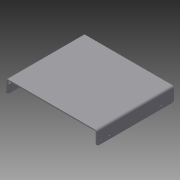
# Autodesk Inventor part: Bed
Saved by Autodesk Inventor 2015 (Build 190159000, 159)
## iProperties
Created: 2015-12-09
Part Number: Bed
Material: Generic
Document SubType Name: Sheet Metal
Designer: Nick
Density: 1 g/cm^3
Flat Pattern Width: 21.3893 cm
Flat Pattern Length: 31.6732 cm
Flat Pattern Area: 677.468 cm^2
Sheet Metal Rule: Default
Sheet Metal Width: 8.421 in
Sheet Metal Length: 12.470 in
Sheet Metal Area: 105.008 in^2
Appearance: Default
Author: Nick
Autodesk Inventor part; units mm, degrees
ref_plane "YZ Plane" through (0, 0, 0) normal (1, 0, 0) x (0, 1, 0)
ref_plane "XZ Plane" through (0, 0, 0) normal (0, 1, 0) x (-1, 0, 0)
ref_plane "XY Plane" through (0, 0, 0) normal (0, 0, 1) x (1, 0, 0)
sketch "Sketch1" plane through (0, 0, 0) normal (0, 1, 0) x (-1, 0, 0)
  line L0 (0, 0) -> (0, -213.8934)
  line L1 (0, -213.8934) -> (236.982, -213.8934)
  line L2 (236.982, -213.8934) -> (236.982, 0)
  line L3 (236.982, 0) -> (0, 0)
  line L4 (246.3292, 0) -> (270.5069, 0)
  line L5 (246.3292, -213.8934) -> (246.3292, 0)
  line L6 (270.5069, 0) -> (270.5069, 0)
  line L7 (276.8569, -6.35) -> (276.8569, -207.5434)
  arc A0 (276.8569, -6.35) -> (270.5069, 0) centre (270.5069, -6.35) ccw
  arc A1 (270.5068, -213.8934) -> (276.8569, -207.5434) centre (270.5069, -207.5434) ccw
  line L8 (236.982, 0) -> (246.3292, 0)
  line L9 (236.982, -213.8934) -> (246.3292, -213.8934)
  line L10 (241.6556, 0) -> (241.6556, -213.8934)
  line L11 (246.3292, -213.8934) -> (270.5068, -213.8934)
  line L12 (118.491, 0) -> (118.491, -213.8934)
  line L13 (0, -213.8934) -> (0, 0)
  line L14 (-9.3472, 0) -> (-33.5249, 0)
  line L15 (-9.3472, -213.8934) -> (-9.3472, 0)
  line L16 (-33.5249, 0) -> (-33.5249, 0)
  line L17 (-39.8749, -6.35) -> (-39.8749, -207.5434)
  arc A2 (-33.5249, 0) -> (-39.8749, -6.35) centre (-33.5249, -6.35) ccw
  arc A3 (-39.8749, -207.5434) -> (-33.5248, -213.8934) centre (-33.5249, -207.5434) ccw
  line L18 (0, 0) -> (-9.3472, 0)
  line L19 (0, -213.8934) -> (-9.3472, -213.8934)
  line L20 (-4.6736, 0) -> (-4.6736, -213.8934)
  line L21 (-9.3472, -213.8934) -> (-33.5248, -213.8934)
  circle A4 centre (267.6621, -35.1028) radius 1.4986
  line L22 (276.8569, -106.9467) -> (236.982, -106.9467)
  circle A5 centre (267.6621, -178.7906) radius 1.4986
  circle A6 centre (-30.6801, -35.1028) radius 1.4986
  circle A7 centre (-30.6801, -178.7906) radius 1.4986
  line L23 (246.9642, -4.4704) -> (249.3518, -4.4704)
  line L24 (249.3518, -4.4704) -> (249.3518, -10.6934)
  line L25 (249.3518, -10.6934) -> (246.9642, -10.6934)
  line L26 (246.9642, -10.6934) -> (246.9642, -4.4704)
  line L27 (249.3518, -4.4704) -> (251.5616, -4.4704)
  line L28 (251.5616, -4.4704) -> (251.5616, -10.6934)
  line L29 (251.5616, -10.6934) -> (253.9492, -10.6934)
  line L30 (253.9492, -10.6934) -> (253.9492, -4.4704)
  line L31 (253.9492, -4.4704) -> (251.5616, -4.4704)
  line L32 (-26.0096, -2.9972) -> (-34.4424, -2.9972)
  line L33 (-34.4424, -2.9972) -> (-34.4424, -4.9276)
  line L34 (-34.4424, -4.9276) -> (-26.0096, -4.9276)
  line L35 (-26.0096, -4.9276) -> (-26.0096, -2.9972)
  line L36 (-34.4424, -10.287) -> (-26.0096, -10.287)
  line L37 (-34.4424, -10.287) -> (-34.4424, -12.2174)
  line L38 (-34.4424, -12.2174) -> (-26.0096, -12.2174)
  line L39 (-26.0096, -12.2174) -> (-26.0096, -10.287)
  point P0 (276.8569, 0)
  point P1 (-39.8749, 0)
  dimension "d1" = 213.8934
  dimension "d2" = 236.982
  dimension "d3" = 24.1776
  dimension "d4" = 6.35
  dimension "d5" = 6.35
  dimension "d6" = 9.3472
  dimension "d7" = 213.8934
  dimension "d8" = 24.1776
  dimension "d11" = 2.9972
  dimension "d12" = 9.1948
  dimension "d13" = 35.1028
  dimension "d14" = 4.4704
  dimension "d15" = 6.223
  dimension "d16" = 2.3876
  dimension "d17" = 0.635
  dimension "d18" = 2.2098
  dimension "d19" = 2.3876
  dimension "d20" = 6.223
  dimension "d21" = 16.6624
  dimension "d22" = 8.4328
  dimension "d23" = 2.9972
  dimension "d24" = 1.9304
  dimension "d25" = 5.3594
  dimension "d26" = 1.9304
  dimension "d27" = 8.4328
  dimension "d28" = 5.4325
  measures "d1" distance of L0.start L0.end
  measures "d2" distance of L0.end L1.end
  measures "d3" distance of L4.start L4.end
  measures "d4" distance of L4.end point (276.857, 0)
  measures "d5" radius of A0
  measures "d6" distance of L2.end L4.start
  measures "d7" distance of L5.start L4.start
  measures "d8" distance of L5.start L11.end
  measures "d11" diameter of A4
  measures "d12" distance from line of L7 A4.centre
  measures "d13" distance from line of L4 A4.centre
  measures "d14" distance between parallel lines of L23 L4
  measures "d15" distance between parallel lines of L25 L23
  measures "d16" distance between parallel lines of L24 L26
  measures "d17" distance from line of L4.start L26
  measures "d18" distance of L23.end L27.end
  measures "d19" distance of L28.end L29.end
  measures "d20" distance of L29.end L30.end
  measures "d21" distance from line of L14.start L35
  measures "d22" distance between parallel lines of L33 L35
  measures "d23" distance between parallel lines of L14 L32
  measures "d24" distance between parallel lines of L34 L32
  measures "d25" distance between parallel lines of L34 L36
  measures "d26" distance of L36.start L37.end
  measures "d27" distance of L37.end L38.end
  measures "d28" distance between parallel lines of L17 L37
extrude "Plate1" add sketch "Sketch1" along normal blind 3.048
sketch "Sketch2" plane through (0, 0, 0) normal (0, -1, 0) x (1, 0, 0)
  line L0 (4.6736, 0) -> (4.6736, -213.8934) projected
  line L1 (-241.6556, 0) -> (-241.6556, -213.8934) projected
  line L2 (4.6736, 0) -> (4.6736, -213.8934)
  line L3 (33.5249, 0) -> (-270.5069, 0) projected
  line L4 (-241.6556, 0) -> (-241.6556, -213.8934)
  line L5 (33.5248, -213.8934) -> (-270.5068, -213.8934) projected
  point P0 (0, 0)
  constraints: 4 end point, 2 perpendicular
fold "Fold1" angle 90 bend radius 3.048 thickness 3.048 k factor 0.44 line from (4.6736, 0, 0) to (4.6736, 0, -213.8934) line at bend centre moving side (1, 0, 0) folds toward (0, -1, 0)
fold "Fold2" angle 90 bend radius 3.048 thickness 3.048 k factor 0.44 line from (-241.6556, 0, 0) to (-241.6556, 0, -213.8934) line at bend centre moving side (-1, 0, 0) folds toward (0, -1, 0)
equation "\"d30\" = BendReliefWidth"
equation "\"d31\" = BendReliefDepth"
equation "\"d32\" = MinimumRemnant"
equation "\"d33\" = BendRadius"
equation "\"d35\" = BendRadius"
equation "\"d36\" = BendReliefWidth"
equation "\"d37\" = BendReliefDepth"
equation "\"d38\" = MinimumRemnant"
equation "\"d39\" = BendRadius"
equation "\"d41\" = BendRadius"
equation "\"BendRadius\" = Thickness"
equation "\"BendReliefWidth\" = Thickness"
equation "\"BendReliefDepth\" = 0.5 * Thickness"
equation "\"CornerReliefSize\" = 4 * Thickness"
equation "\"MinimumRemnant\" = 2 * Thickness"
equation "\"TransitionRadius\" = BendRadius"
equation "\"JacobiRadiusSize\" = BendRadius"
equation "\"GapSize\" = Thickness"
equation "\"d29\" = BendRadius"
equation "\"Thickness\" = 3.048"
body "Solid1"
